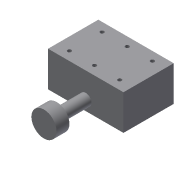
# Autodesk Inventor part: 00_Z-stage
Saved by Autodesk Inventor 2019.4 (Build 234330000, 330)
## iProperties
Created: 2020-11-13
Part Number: 00_Z-stage
Material: Generic
Document SubType Name: Modeling
Designer: diederichbenedict
Density: 1 g/cm^3
Appearance: Default
Author: diederichbenedict
Autodesk Inventor part; units mm, degrees
ref_plane "YZ Plane" through (0, 0, 0) normal (1, 0, 0) x (0, 1, 0)
ref_plane "XZ Plane" through (0, 0, 0) normal (0, 1, 0) x (-1, 0, 0)
ref_plane "XY Plane" through (0, 0, 0) normal (0, 0, 1) x (1, 0, 0)
sketch "Sketch1" plane through (0, 0, 0) normal (0, 1, 0) x (-1, 0, 0)
  line L0 (0, 0) -> (60, 0)
  line L1 (60, 0) -> (60, -40)
  line L2 (60, -40) -> (0, -40)
  line L3 (0, -40) -> (0, 0)
  dimension "d0" = 60
  dimension "d1" = 40
  constraints: 8 end point, 2 parallel, 1 horizontal, 1 perpendicular
  measures "d0" distance of L1.end L2.end
  measures "d1" distance of L0.end L1.end
extrude "Extrusion1" add sketch "Sketch1" along normal blind 28
sketch "Sketch2" plane through (-60, 0, 0) normal (0, 0, 1) x (1, 0, 0)
  circle A0 centre (30, 8) radius 4.6
  line L0 (60, 0) -> (60, 28) projected
  line L1 (60, 0) -> (0, 0) projected
  dimension "d4" = 9.2
  dimension "d5" = 30
  dimension "d6" = 8
  constraints: 1 centre point
  measures "d4" diameter of A0
  measures "d5" distance from line of A0.centre L0
  measures "d6" distance from line of A0.centre L1
extrude "Extrusion2" add sketch "Sketch2" along normal blind 23
sketch "Sketch3" plane through (-30, 8, 23) normal (0, 0, 1) x (1, 0, 0)
  circle A0 centre (0, 0) radius 4.6 projected
  circle A1 centre (0, -0.2633) radius 10
  point P0 (30, -8)
  dimension "d9" = 20
  constraints: 1 centre point
  measures "d9" diameter of A1
extrude "Extrusion3" add sketch "Sketch3" along normal blind 10.25 contours A0 | A1
sketch "Sketch4" plane through (0, 0, 0) normal (0, -1, 0) x (1, 0, 0)
  line L0 (0, 0) -> (-60, 0) projected
  line L1 (-60, 0) -> (-60, -40) projected
  line L2 (-60, -40) -> (0, -40) projected
  line L3 (0, -40) -> (0, 0) projected
  line L4 (-45, -35) -> (-15, -35)
  line L5 (-15, -35) -> (-15, -5)
  line L6 (-15, -5) -> (-45, -5)
  line L7 (-45, -5) -> (-45, -35)
  line L8 (-45, -35) -> (-15, -5) construction
  line L9 (-15, -35) -> (-45, -5) construction
  point P0 (-30, -20)
  dimension "d12" = 30
  dimension "d13" = 30
  constraints: 12 end point, 2 midpoint, 2 parallel, 1 horizontal, 1 perpendicular
  measures "d12" distance of L6.end L5.end
  measures "d13" distance of L5.end L4.end
hole "Hole1" at (-15, 0, -5) at (-15, 0, -35) at (-45, 0, -35) at (-45, 0, -5) direction (0, 1, 0) diameter 3 depth 8 tip angle 118
sketch "Sketch5" plane through (0, 28, 0) normal (0, 1, 0) x (1, 0, 0)
  line L0 (-60, 0) -> (0, 0) projected
  line L1 (0, 0) -> (0, 40) projected
  line L2 (0, 40) -> (-60, 40) projected
  line L3 (-60, 40) -> (-60, 0) projected
  line L4 (-10, 7) -> (-50, 7)
  line L5 (-50, 7) -> (-50, 33)
  line L6 (-50, 33) -> (-10, 33)
  line L7 (-10, 33) -> (-10, 7)
  line L8 (-10, 7) -> (-50, 33) construction
  line L9 (-50, 7) -> (-10, 33) construction
  point P0 (-30, 20)
  point P1 (-30, 7)
  point P2 (-30, 33)
  dimension "d21" = 40
  dimension "d22" = 26
  constraints: 12 end point, 4 midpoint, 2 parallel, 1 horizontal, 1 perpendicular
  measures "d21" distance of L5.end L6.end
  measures "d22" distance of L4.end L5.end
hole "Hole2" at (-30, 28, -7) at (-30, 28, -33) at (-50, 28, -7) at (-50, 28, -33) at (-10, 28, -33) at (-10, 28, -7) direction (0, -1, 0) diameter 3 depth 8 tip angle 118
body "Solid1"
